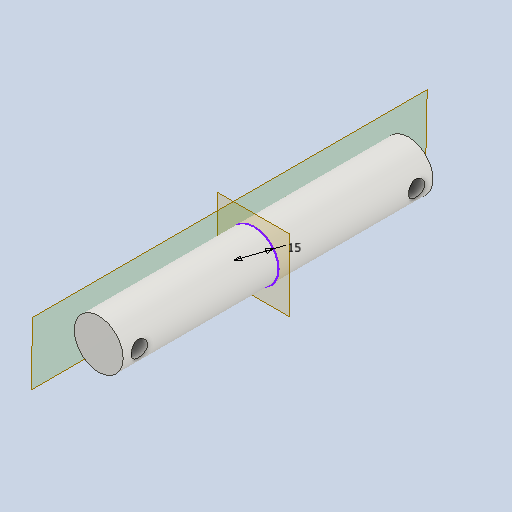
# Autodesk Inventor part: rotating axel
Saved by Autodesk Inventor 2022.2 (Build 262287010, 287A)
## iProperties
Created: 2022-04-06
Part Number: rotating axel
Material: Steel, Mild
Document SubType Name: Modeling
Designer: Finn Oriwohl
Mass: 124.849 g
Surface Area: 45.9458 cm^2
Volume: 15.9043 cm^3
Density: 7.85 g/cm^3
Appearance: Steel
Author: Finn Oriwohl
Autodesk Inventor part; units mm, degrees
ref_plane "YZ Plane" through (0, 0, 0) normal (1, 0, 0) x (0, 1, 0)
ref_plane "XZ Plane" through (0, 0, 0) normal (0, 1, 0) x (-1, 0, 0)
ref_plane "XY Plane" through (0, 0, 0) normal (0, 0, 1) x (1, 0, 0)
ref_plane "Work Plane6" through (81.3851, 174.1567, 420.1401) normal (0, 0, 1) x (1, 0, 0)
sketch "Sketch1" plane through (81.3851, 174.1567, 420.1401) normal (0, 0, 1) x (1, 0, 0)
  circle A0 centre (0, 0) radius 7.5
  dimension "d0" = 15
  constraints: 1 centre point
  measures "d0" diameter of A0
extrude "Extrusion1" add sketch "Sketch1" along normal mid plane 95
ref_plane "Work Plane8" through (73.8871, 174.3299, 420.1401) normal (-0.9997333, 0.0230925, 0) x (0, 0, -1)
ref_plane "Work Plane7" through (124.4226, 218.5866, 522.8067) normal (-0.9997333, 0.0230925, 0) x (0, 0, -1)
sketch "Sketch2" plane through (73.8871, 174.3299, 420.1401) normal (-0.9997333, 0.0230925, 0) x (0, 0, -1)
  circle A0 centre (42.5, 0.0019) radius 2.5
  line L0 (-31.3742, -0.0013) -> (-31.3742, -8.6263) construction
  line L1 (0, 0) -> (0, -5.2726) construction
  circle A1 centre (-42.5, 0.0019) radius 2.5
  line L2 (40, 9.5) -> (40, -9.5) projected
  line L3 (47.5, -7.5) -> (47.5, 7.5) projected
  point P0 (420.1401, 175.9896)
  dimension "d5" = 5
  dimension "d7" = 5
  constraints: 4 end point, 2 centre point, 2 vertical, 1 symmetric about line, 1 tangent, 1 other
  measures "d5" diameter of A0
  measures "d7" distance from line of L3 A0.centre
extrude "Extrusion3" cut sketch "Sketch2" against normal through all
body "Solid1"
